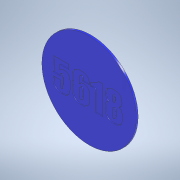
# Autodesk Inventor part: Blue Alliance Marker 5618
Saved by Autodesk Inventor 2022 (Build 260153000, 153)
## iProperties
Created: 2022-11-08
Part Number: Blue Alliance Marker 5618
Material: Generic
Document SubType Name: Modeling
Designer: matt
Density: 1 g/cm^3
Appearance: Default
Author: matt
Autodesk Inventor part; units mm, degrees
ref_plane "YZ Plane" through (0, 0, 0) normal (1, 0, 0) x (0, 1, 0)
ref_plane "XZ Plane" through (0, 0, 0) normal (0, 1, 0) x (-1, 0, 0)
ref_plane "XY Plane" through (0, 0, 0) normal (0, 0, 1) x (1, 0, 0)
sketch "Sketch1" plane through (0, 0, 0) normal (0, 0, 1) x (1, 0, 0)
  circle A0 centre (0, 0) radius 31.75
  line L0 (-24.9602, 8.8198) -> (23.1368, 8.8198) construction
  line L1 (23.1368, 8.8198) -> (23.1368, -14.9885) construction
  line L2 (23.1368, -14.9885) -> (-24.9602, -14.9885) construction
  line L3 (-24.9602, -14.9885) -> (-24.9602, 8.8198) construction
  line L4 (-13.7341, 8.4322) -> (-13.7341, 5.3888)
  line L5 (-13.7341, 5.3888) -> (-19.6343, 5.3888)
  line L6 (-19.6343, 5.3888) -> (-19.6343, 2.1444)
  spline S0 degree 2 poles (-19.6343, 2.1444) (-18.5289, 3.4507) (-16.7775, 3.4507) knots 0 0 0 1 1 1
  spline S1 degree 2 poles (-16.7775, 3.4507) (-14.8107, 3.4507) (-12.8009, 1.2543) (-12.8009, -1.8752) knots 0 0 0 1 2 2 2
  line L7 (-12.8009, -1.8752) -> (-12.8009, -4.5884)
  spline S2 degree 2 poles (-12.8009, -4.5884) (-12.8009, -6.6126) (-13.1886, -8.5076) (-14.4662, -10.1154) (-16.7344, -10.9767) (-18.371, -10.9767) knots 0 0 0 1 2 3 4 4 4
  spline S3 degree 2 poles (-18.371, -10.9767) (-20.2085, -10.9767) (-23.0078, -9.6991) (-24.185, -7.1581) (-24.185, -4.5023) knots 0 0 0 1 2 3 3 3
  line L8 (-24.185, -4.5023) -> (-24.185, -3.4687)
  line L9 (-24.185, -3.4687) -> (-19.4333, -3.4687)
  line L10 (-19.4333, -3.4687) -> (-19.4333, -4.6602)
  spline S4 degree 2 poles (-19.4333, -4.6602) (-19.4333, -6.4978) (-19.1749, -8.0482) (-18.3997, -8.0482) knots 0 0 0 1 2 2 2
  spline S5 degree 2 poles (-18.3997, -8.0482) (-18.0551, -8.0482) (-17.6101, -7.6031) (-17.5814, -7.0863) (-17.5527, -5.0909) knots 0 0 0 1 2 3 3 3
  line L11 (-17.5527, -5.0909) -> (-17.5527, -1.3297)
  spline S6 degree 2 poles (-17.5527, -1.3297) (-17.5527, -0.253) (-17.9977, 0.5222) (-18.5289, 0.5222) knots 0 0 0 1 2 2 2
  spline S7 degree 2 poles (-18.5289, 0.5222) (-18.859, 0.5222) (-19.3041, 0.1202) (-19.4333, -0.3392) (-19.4333, -1.1718) knots 0 0 0 1 2 3 3 3
  line L12 (-19.4333, -1.1718) -> (-24.1419, -1.1718)
  line L13 (-24.1419, -1.1718) -> (-23.941, 8.4322)
  line L14 (-23.941, 8.4322) -> (-13.7341, 8.4322)
  line L15 (0.234, 3.379) -> (-4.5177, 3.379)
  spline S8 degree 2 poles (-4.5177, 3.379) (-4.5177, 4.714) (-4.5751, 5.4031) (-5.0776, 5.8768) (-5.5226, 5.8768) knots 0 0 0 1 2 3 3 3
  spline S9 degree 2 poles (-5.5226, 5.8768) (-5.8815, 5.8768) (-6.3552, 5.4318) (-6.427, 4.7284) (-6.427, 3.6517) knots 0 0 0 1 2 3 3 3
  line L16 (-6.427, 3.6517) -> (-6.427, 0.6083)
  spline S10 degree 2 poles (-6.427, 0.6083) (-6.0681, 1.3835) (-4.6469, 2.1444) (-3.6133, 2.1444) knots 0 0 0 1 2 2 2
  spline S11 degree 2 poles (-3.6133, 2.1444) (-2.3069, 2.1444) (-0.3115, 0.7375) (0.234, -1.2436) (0.234, -2.9232) knots 0 0 0 1 2 3 3 3
  line L17 (0.234, -2.9232) -> (0.234, -4.4449)
  spline S12 degree 2 poles (0.234, -4.4449) (0.234, -6.4403) (-0.0675, -8.3927) (-1.4025, -10.058) (-3.7138, -10.9767) (-5.2642, -10.9767) knots 0 0 0 1 2 3 4 4 4
  spline S13 degree 2 poles (-5.2642, -10.9767) (-7.1735, -10.9767) (-9.6283, -9.9144) (-10.9491, -7.9333) (-11.1788, -5.7369) (-11.1788, -2.5787) knots 0 0 0 1 2 3 4 4 4
  line L18 (-11.1788, -2.5787) -> (-11.1788, 0.0484)
  spline S14 degree 2 poles (-11.1788, 0.0484) (-11.1788, 3.4507) (-10.9778, 5.7476) (-9.5422, 7.8005) (-7.0587, 8.8198) (-5.4365, 8.8198) knots 0 0 0 1 2 3 4 4 4
  spline S15 degree 2 poles (-5.4365, 8.8198) (-3.441, 8.8198) (-0.8714, 7.5278) (0.234, 5.1734) (0.234, 3.379) knots 0 0 0 1 2 3 3 3
  spline S16 degree 2 poles (-4.5177, -2.5643) (-4.5177, -1.545) (-4.9627, -0.7985) (-5.4652, -0.7985) knots 0 0 0 1 2 2 2
  spline S17 degree 2 poles (-5.4652, -0.7985) (-5.9676, -0.7985) (-6.427, -1.5163) (-6.427, -2.5643) knots 0 0 0 1 2 2 2
  line L19 (-6.427, -2.5643) -> (-6.427, -6.0097)
  spline S18 degree 2 poles (-6.427, -6.0097) (-6.427, -7.273) (-5.9964, -8.0482) (-5.4795, -8.0482) knots 0 0 0 1 2 2 2
  spline S19 degree 2 poles (-5.4795, -8.0482) (-5.1781, -8.0482) (-4.5177, -7.4452) (-4.5177, -6.1245) knots 0 0 0 1 2 2 2
  line L20 (-4.5177, -6.1245) -> (-4.5177, -2.5643)
  line L21 (9.192, 8.4322) -> (9.192, -10.6178)
  line L22 (9.192, -10.6178) -> (4.4402, -10.6178)
  line L23 (4.4402, -10.6178) -> (4.4402, -0.3966)
  spline S20 degree 2 poles (4.4402, -0.3966) (4.4402, 1.8142) (4.2249, 2.7042) (3.2774, 3.1636) (1.6409, 3.1636) knots 0 0 0 1 2 3 3 3
  line L24 (1.6409, 3.1636) -> (1.1671, 3.1636)
  line L25 (1.1671, 3.1636) -> (1.1671, 5.3888)
  spline S21 degree 2 poles (1.1671, 5.3888) (4.6125, 6.1209) (6.407, 8.4322) knots 0 0 0 1 1 1
  line L26 (6.407, 8.4322) -> (9.192, 8.4322)
  spline S22 degree 2 poles (20.1166, 0.2064) (21.1646, -0.2243) (22.2987, -1.9039) (22.2987, -5.0765) knots 0 0 0 1 2 2 2
  spline S23 degree 2 poles (22.2987, -5.0765) (22.2987, -7.3878) (21.4087, -9.5699) (18.8103, -10.9767) (16.6426, -10.9767) knots 0 0 0 1 2 3 3 3
  spline S24 degree 2 poles (16.6426, -10.9767) (14.5179, -10.9767) (12.0487, -9.6273) (10.9721, -7.4165) (10.9721, -4.8469) knots 0 0 0 1 2 3 3 3
  spline S25 degree 2 poles (10.9721, -4.8469) (10.9721, -3.1098) (11.5032, -0.5689) (12.9101, 0.2064) knots 0 0 0 1 2 2 2
  spline S26 degree 2 poles (12.9101, 0.2064) (12.02, 0.6227) (11.1443, 2.4746) (11.1443, 3.8958) knots 0 0 0 1 2 2 2
  spline S27 degree 2 poles (11.1443, 3.8958) (11.1443, 6.3506) (13.8719, 8.8054) (16.5851, 8.8054) knots 0 0 0 1 2 2 2
  spline S28 degree 2 poles (16.5851, 8.8054) (19.729, 8.8054) (22.1264, 6.1927) (22.1264, 3.7666) knots 0 0 0 1 2 2 2
  spline S29 degree 2 poles (22.1264, 3.7666) (22.1264, 2.2305) (21.3369, 0.8667) (20.1166, 0.2064) knots 0 0 0 1 2 2 2
  spline S30 degree 2 poles (17.547, -3.6266) (17.547, -2.5356) (17.102, -1.8178) (16.6139, -1.8178) knots 0 0 0 1 2 2 2
  spline S31 degree 2 poles (16.6139, -1.8178) (16.1401, -1.8178) (15.7238, -2.5069) (15.7238, -3.6266) knots 0 0 0 1 2 2 2
  line L27 (15.7238, -3.6266) -> (15.7238, -6.1102)
  spline S32 degree 2 poles (15.7238, -6.1102) (15.7238, -7.3447) (16.1832, -8.0482) (16.6856, -8.0482) knots 0 0 0 1 2 2 2
  spline S33 degree 2 poles (16.6856, -8.0482) (17.1881, -8.0482) (17.547, -7.3304) (17.547, -6.0671) knots 0 0 0 1 2 2 2
  line L28 (17.547, -6.0671) -> (17.547, -3.6266)
  spline S34 degree 2 poles (17.4465, 4.2834) (17.4465, 5.2596) (17.102, 5.8768) (16.6282, 5.8768) knots 0 0 0 1 2 2 2
  spline S35 degree 2 poles (16.6282, 5.8768) (16.1545, 5.8768) (15.8243, 5.2021) (15.8243, 4.2834) knots 0 0 0 1 2 2 2
  line L29 (15.8243, 4.2834) -> (15.8243, 2.8478)
  spline S36 degree 2 poles (15.8243, 2.8478) (15.8243, 1.9865) (16.1975, 1.3261) (16.6426, 1.3261) knots 0 0 0 1 2 2 2
  spline S37 degree 2 poles (16.6426, 1.3261) (17.1163, 1.3261) (17.4465, 1.9721) (17.4465, 2.9914) knots 0 0 0 1 2 2 2
  line L30 (17.4465, 2.9914) -> (17.4465, 4.2834)
  dimension "d0" = 63.5
  constraints: 1 centre point, 1 coincident, 2 other
  measures "d0" diameter of A0
extrude "Extrusion1" add sketch "Sketch1" along normal blind 1.2 contours A0 | L4 L5 L6 S0 S1 L7 S2 S3 L8 L9 L10 S4 S5 L11 S6 S7 L12 L13 L14 | L15 S8 S9 L16 S10 S11 L17 S12 S13 L18 S14 S15 | L20 S19 S18 L19 S17 S16 | L21 L22 L23 S20 L24 L25 S21 L26 | S22 S23 S24 S25 S26 S27 S28 S29 | L28 S33 S32 L27 S31 S30 | L30 S37 S36 L29 S35 S34
extrude "Extrusion2" cut sketch "Sketch1" against normal blind 0.6 from surface at 1.2 contours L4 L5 L6 S0 S1 L7 S2 S3 L8 L9 L10 S4 S5 L11 S6 S7 L12 L13 L14 | L15 S8 S9 L16 S10 S11 L17 S12 S13 L18 S14 S15 | L21 L22 L23 S20 L24 L25 S21 L26 | S22 S23 S24 S25 S26 S27 S28 S29
body "Solid1"
